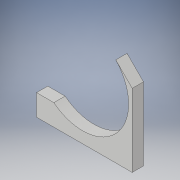
# Autodesk Inventor part: main prototype
Saved by Autodesk Inventor 2018 (Build 220112000, 112)
## iProperties
Created: 2020-01-10
Part Number: main prototype
Material: Generic
Document SubType Name: Modeling
Designer: s-2513225
Density: 1 g/cm^3
Appearance: Default
Author: s-2513225
Autodesk Inventor part; units mm, degrees
ref_plane "YZ Plane" through (0, 0, 0) normal (1, 0, 0) x (0, 1, 0)
ref_plane "XZ Plane" through (0, 0, 0) normal (0, 1, 0) x (-1, 0, 0)
ref_plane "XY Plane" through (0, 0, 0) normal (0, 0, 1) x (1, 0, 0)
sketch "Sketch1" plane through (0, 0, 0) normal (0, 0, 1) x (1, 0, 0)
  circle A0 centre (0, 0) radius 207.9625
  line L0 (-215.7457, 231.7761) -> (224.1521, 231.7761) construction
  line L1 (224.1521, 231.7761) -> (224.1521, -258.7625) construction
  line L2 (224.1521, -258.7625) -> (-207.6479, -258.7625) construction
  line L3 (0, 0) -> (294.0459, 0) construction
  line L4 (294.0459, 0) -> (62.2698, 231.7761) construction
  line L5 (294.0459, 0) -> (621.8269, 0) construction
  line L6 (-129.4556, -162.7564) -> (-480.3051, -162.7564) construction
  line L7 (-480.3051, -162.7564) -> (-480.3051, 0) construction
  line L8 (-480.3051, 0) -> (-129.4556, 0) construction
  line L9 (-129.4556, 0) -> (-129.4556, -162.7564) construction
  line L10 (62.2698, 231.7761) -> (294.0459, 0) construction
  line L11 (294.0459, 0) -> (599.7721, 305.7262)
  line L12 (599.7721, 305.7262) -> (367.996, 537.5023)
  line L13 (367.996, 537.5023) -> (62.2698, 231.7761)
  line L14 (-207.6479, -162.7564) -> (-207.6479, -258.7625)
  line L15 (-207.6479, -258.7625) -> (224.1521, -258.7625)
  line L16 (224.1521, -258.7625) -> (224.1521, 69.8938)
  line L17 (224.1521, 69.8938) -> (149.9298, 144.1161)
  line L18 (-207.6479, -162.7564) -> (-129.4556, -162.7564)
  line L19 (-207.6479, -258.7625) -> (-207.6479, -162.7564) construction
  line L20 (-215.7457, 0) -> (-215.7457, 231.7761) construction
  line L21 (0, -207.9625) -> (0, -258.7625)
  point P0 (-207.9625, 0)
  dimension "d0" = 415.925
  dimension "d3" = 135
  dimension "d6" = 431.8
  dimension "d7" = 50.8
  constraints: 44 end point, 8 parallel, 8 point on line, 5 perpendicular, 4 collinear, 4 point on circle, 3 horizontal, 1 centre point, 1 coincident, 1 equal length
  measures "d0" diameter of A0
  measures "d3" angle of L5 L4
  measures "d6" distance of L1.end L2.end
  measures "d7" distance of L21.start L21.end
extrude "Extrusion1" add sketch "Sketch1" along normal blind 50.8 contours A0 L17 L16 L15 L21 | L21 L15 L14 L18 A0
body "Solid1"
